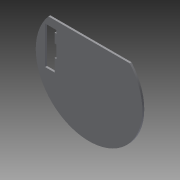
# Autodesk Inventor part: BasePlate
Saved by Autodesk Inventor 2015 (Build 190159000, 159)
## iProperties
Created: 2014-08-15
Part Number: BasePlate
Material: Generic
Document SubType Name: Modeling
Designer: karl
Density: 1 g/cm^3
Appearance: Default
Author: karl
Autodesk Inventor part; units mm, degrees
ref_plane "YZ Plane" through (0, 0, 0) normal (1, 0, 0) x (0, 1, 0)
ref_plane "XZ Plane" through (0, 0, 0) normal (0, 1, 0) x (-1, 0, 0)
ref_plane "XY Plane" through (0, 0, 0) normal (0, 0, 1) x (1, 0, 0)
sketch "Sketch1" plane through (0, 0, 0) normal (0, 1, 0) x (-1, 0, 0)
  circle A0 centre (0, 0) radius 85
  line L0 (-64.8074, 55) -> (64.8074, 55)
  dimension "d0" = 170
  dimension "d1" = 55
  constraints: 2 end point, 2 point on circle, 1 centre point, 1 coincident, 1 horizontal
  measures "d0" diameter of A0
  measures "d1" distance from line of point (0, 0) L0
extrude "Extrusion1" add sketch "Sketch1" along normal blind 3 contours A0 L0 picked at (-1.5877, 8.3779)
sketch "Sketch2" plane through (0, 3, 0) normal (0, 1, 0) x (1, 0, 0)
  line L0 (-75, 25) -> (-60, 25)
  line L1 (-60, 25) -> (-60, -35)
  line L2 (-60, -35) -> (-75, -35)
  line L3 (-75, -35) -> (-75, 25)
  line L4 (-75, -5) -> (-60, -5) construction
  point P0 (0, 0)
  dimension "d4" = 15
  dimension "d5" = 60
  dimension "d6" = 60
  dimension "d7" = 5
  constraints: 10 end point, 2 midpoint, 2 parallel, 1 horizontal, 1 perpendicular
  measures "d4" distance of L1.end L2.end
  measures "d5" distance of L0.end L1.end
  measures "d6" distance from line of point (0, 0) L1
  measures "d7" distance from line of point (0, 0) L4
extrude "Extrusion2" cut sketch "Sketch2" against normal blind 3
sketch "Sketch3" plane through (0, 3, 0) normal (0, 1, 0) x (1, 0, 0)
  line L0 (-60, -35) -> (-60, 25) projected
  line L1 (-60, -15) -> (-57, -15)
  line L2 (-57, -15) -> (-57, 5)
  line L3 (-57, 5) -> (-60, 5)
  line L4 (-60, 5) -> (-60, -15)
  line L5 (-60, -35) -> (-57, -35)
  line L6 (-57, -35) -> (-57, -30)
  line L7 (-57, -30) -> (-60, -30)
  line L8 (-60, -30) -> (-60, -35)
  point P0 (0, 0)
  point P1 (-57, -5)
  point P2 (-60, -5)
  dimension "d10" = 3
  dimension "d11" = 20
  dimension "d12" = 3
  dimension "d13" = 5
  dimension "d14" = 15
  constraints: 16 end point, 4 parallel, 2 horizontal, 2 midpoint, 2 perpendicular, 1 collinear, 1 horizontal alignment, 1 point on line
  measures "d10" distance of L3.end L2.end
  measures "d11" distance of L2.end L1.end
  measures "d12" distance of L7.end L6.end
  measures "d13" distance of L6.end L5.end
  measures "d14" distance from line of L7 L1.start
extrude "Extrusion3" cut sketch "Sketch3" against normal blind 3
sketch "Sketch8" plane through (0, 3, 0) normal (0, 1, 0) x (1, 0, 0)
  line L0 (-10, -13) -> (-50, -13) construction
  line L1 (-10, -11.5) -> (-50, -11.5)
  line L2 (-50, -14.5) -> (-10, -14.5)
  arc A0 (-10, -14.5) -> (-10, -11.5) centre (-10, -13) ccw
  arc A1 (-50, -11.5) -> (-50, -14.5) centre (-50, -13) ccw
  line L3 (-10, -5) -> (-50, -5) construction
  line L4 (-10, -3.5) -> (-50, -3.5)
  line L5 (-50, -6.5) -> (-10, -6.5)
  arc A2 (-10, -6.5) -> (-10, -3.5) centre (-10, -5) ccw
  arc A3 (-50, -3.5) -> (-50, -6.5) centre (-50, -5) ccw
  line L6 (-10, 3) -> (-50, 3) construction
  line L7 (-10, 4.5) -> (-50, 4.5)
  line L8 (-50, 1.5) -> (-10, 1.5)
  arc A4 (-10, 1.5) -> (-10, 4.5) centre (-10, 3) ccw
  arc A5 (-50, 4.5) -> (-50, 1.5) centre (-50, 3) ccw
  point P0 (0, 0)
  point P1 (-30, -13)
  point P2 (-30, -5)
  point P3 (-30, 3)
  dimension "d54" = 3
  dimension "d55" = 3
  dimension "d56" = 3
  dimension "d57" = 5
  dimension "d58" = 5
  dimension "d59" = 5
  dimension "d60" = 40
  dimension "d61" = 30
  constraints: 24 end point, 12 point on circle, 12 tangent, 7 parallel, 6 centre point, 3 midpoint, 2 vertical alignment, 1 horizontal
  measures "d54" diameter of A1
  measures "d55" diameter of A3
  measures "d56" diameter of A5
  measures "d57" distance between parallel lines of L1 L5
  measures "d58" distance between parallel lines of L8 L4
  measures "d59" distance from line of point (0, 0) L3
  measures "d60" distance of L6.start L6.end
  measures "d61" horizontal distance of point (0, 0) point (-30, -5)
extrude "Extrusion7" cut sketch "Sketch8" against normal blind 3
sketch "Sketch4" plane through (0, 3, 0) normal (0, 1, 0) x (1, 0, 0)
  line L0 (-60, -55) -> (-40, -55)
  line L1 (-40, -55) -> (-40, -52)
  line L2 (-40, -52) -> (-60, -52)
  line L3 (-60, -52) -> (-60, -55)
  line L4 (-64.8074, -55) -> (64.8074, -55) projected
  line L5 (-20, -55) -> (-10, -55)
  line L6 (-10, -55) -> (-10, -52)
  line L7 (-10, -52) -> (-20, -52)
  line L8 (-20, -52) -> (-20, -55)
  point P0 (0, 0)
  dimension "d17" = 20
  dimension "d18" = 3
  dimension "d19" = 10
  dimension "d20" = 3
  dimension "d21" = 10
  dimension "d22" = 20
  constraints: 16 end point, 4 parallel, 2 horizontal, 2 perpendicular, 1 collinear, 1 point on line
  measures "d17" distance of L2.end L1.end
  measures "d18" distance of L1.end L0.end
  measures "d19" distance of L7.end L6.end
  measures "d20" distance of L6.end L5.end
  measures "d21" distance from line of L6 point (0, 0)
  measures "d22" distance between parallel lines of L1 L8
extrude "Extrusion4" cut sketch "Sketch4" against normal blind 3
sketch "Sketch5" plane through (0, 0, 0) normal (0, -1, 0) x (1, 0, 0)
  line L0 (-50, 17.5) -> (-30, 17.5)
  line L1 (-30, 17.5) -> (-30, 20.5)
  line L2 (-30, 20.5) -> (-50, 20.5)
  line L3 (-50, 20.5) -> (-50, 17.5)
  line L4 (-10, 17.5) -> (10, 17.5)
  line L5 (10, 17.5) -> (10, 20.5)
  line L6 (10, 20.5) -> (-10, 20.5)
  line L7 (-10, 20.5) -> (-10, 17.5)
  line L8 (30, 17.5) -> (50, 17.5)
  line L9 (50, 17.5) -> (50, 20.5)
  line L10 (50, 20.5) -> (30, 20.5)
  line L11 (30, 20.5) -> (30, 17.5)
  point P0 (0, 0)
  dimension "d25" = 17.5
  dimension "d26" = 3
  dimension "d27" = 30
  dimension "d28" = 20
  dimension "d31" = 40
  constraints: 24 end point, 2 horizontal, 2 parallel, 1 collinear, 1 perpendicular, 15 other
  measures "d25" distance from line of point (0, 0) L0
  measures "d26" distance between parallel lines of L0 L2
  measures "d27" distance from line of point (0, 0) L1
  measures "d28" distance of L1.end L2.end
  measures "d31" distance of L0.start L4.start
extrude "Extrusion5" cut sketch "Sketch5" against normal blind 3
sketch "Sketch6" plane through (0, 3, 0) normal (0, 1, 0) x (1, 0, 0)
  point P0 (0, 0)
sketch "Sketch7" plane through (0, 3, 0) normal (0, 1, 0) x (1, 0, 0)
  line L0 (55, 20) -> (-55, 20) construction
  line L1 (-55, 20) -> (-55, 58) construction
  line L2 (-55, 58) -> (55, 58) construction
  line L3 (55, 58) -> (55, 20) construction
  line L4 (40, 58) -> (20, 58)
  line L5 (20, 58) -> (20, 61)
  line L6 (20, 61) -> (40, 61)
  line L7 (40, 61) -> (40, 58)
  line L8 (-40, 58) -> (-20, 58)
  line L9 (-20, 58) -> (-20, 61)
  line L10 (-20, 61) -> (-40, 61)
  line L11 (-40, 61) -> (-40, 58)
  line L12 (40, 20) -> (20, 20)
  line L13 (20, 20) -> (20, 17)
  line L14 (20, 17) -> (40, 17)
  line L15 (40, 17) -> (40, 20)
  line L16 (-20, 20) -> (-40, 20)
  line L17 (-40, 20) -> (-40, 17)
  line L18 (-40, 17) -> (-20, 17)
  line L19 (-20, 17) -> (-20, 20)
  line L20 (55, 34) -> (58, 34)
  line L21 (58, 34) -> (58, 44)
  line L22 (58, 44) -> (55, 44)
  line L23 (55, 44) -> (55, 34)
  line L24 (-55, 34) -> (-58, 34)
  line L25 (-58, 34) -> (-58, 44)
  line L26 (-58, 44) -> (-55, 44)
  line L27 (-55, 44) -> (-55, 34)
  point P0 (0, 0)
  point P1 (0, 58)
  point P2 (58, 39)
  point P3 (55, 39)
  dimension "d38" = 110
  dimension "d39" = 38
  dimension "d40" = 20
  dimension "d41" = 20
  dimension "d42" = 3
  dimension "d43" = 20
  dimension "d44" = 3
  dimension "d45" = 20
  dimension "d46" = 40
  dimension "d47" = 3
  dimension "d50" = 3
  dimension "d51" = 10
  dimension "d52" = 3
  dimension "d53" = 10
  constraints: 56 end point, 14 parallel, 8 point on line, 7 horizontal, 7 perpendicular, 4 collinear, 3 midpoint, 1 horizontal alignment, 1 vertical alignment
  measures "d38" distance of L1.end L2.end
  measures "d39" distance of L0.end L1.end
  measures "d40" distance from line of point (0, 0) L0
  measures "d41" distance of L5.end L6.end
  measures "d42" distance of L4.end L5.end
  measures "d43" distance of L10.end L9.end
  measures "d44" distance of L9.end L8.end
  measures "d45" distance from line of L9 point (0, 0)
  measures "d46" distance between parallel lines of L9 L5
  measures "d47" distance of L13.end L12.end
  measures "d50" distance of L22.end L21.end
  measures "d51" distance of L21.end L20.end
  measures "d52" distance of L25.end L26.end
  measures "d53" distance of L24.end L25.end
extrude "Extrusion6" cut sketch "Sketch7" against normal blind 3
mirror "Mirror1" about plane through (0, 0, 0) normal (1, 0, 0) of "Extrusion2", "Extrusion3", "Extrusion4", "Extrusion7"
sketch "Sketch9" plane through (0, 3, 0) normal (0, 1, 0) x (1, 0, 0)
  line L0 (1.5, 66) -> (-1.5, 66)
  line L1 (-1.5, 66) -> (-1.5, 76)
  line L2 (-1.5, 76) -> (1.5, 76)
  line L3 (1.5, 76) -> (1.5, 66)
  line L4 (20, 61) -> (40, 61) projected
  point P0 (0, 0)
  point P1 (0, 66)
  dimension "d64" = 3
  dimension "d65" = 10
  dimension "d66" = 5
  constraints: 8 end point, 2 parallel, 1 horizontal, 1 midpoint, 1 perpendicular, 1 vertical alignment
  measures "d64" distance of L1.end L2.end
  measures "d65" distance of L0.end L1.end
  measures "d66" distance from line of point (0, 66) L4
extrude "Extrusion8" cut sketch "Sketch9" against normal blind 3
body "Solid1"
